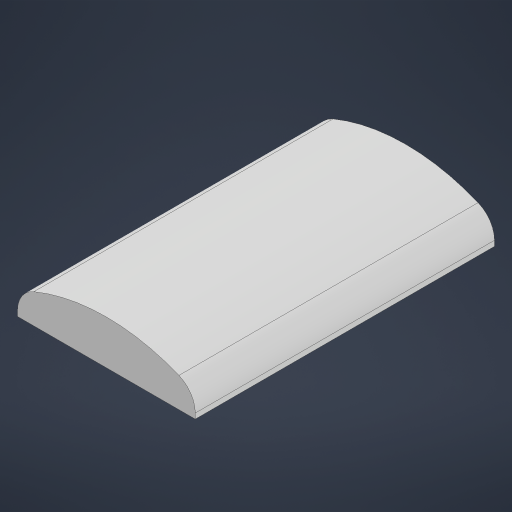
# Autodesk Inventor part: LED-streifen
Saved by Autodesk Inventor 2023 (Build 270158000, 158)
## iProperties
Created: 2022-04-28
Part Number: LED-streifen
Material: Generic
Document SubType Name: Modeling
Designer: Simon
Density: 1 g/cm^3
Appearance: Default
Author: Simon
Autodesk Inventor part; units mm, degrees
ref_plane "YZ Plane" through (0, 0, 0) normal (1, 0, 0) x (0, 1, 0)
ref_plane "XZ Plane" through (0, 0, 0) normal (0, 1, 0) x (-1, 0, 0)
ref_plane "XY Plane" through (0, 0, 0) normal (0, 0, 1) x (1, 0, 0)
sketch "Sketch1" plane through (0, 0, 0) normal (0, 1, 0) x (-1, 0, 0)
  line L0 (5.05, 8.5) -> (-5.05, 8.5)
  line L1 (-5.05, 8.5) -> (-5.05, -8.5)
  line L2 (-5.05, -8.5) -> (5.05, -8.5)
  line L3 (5.05, -8.5) -> (5.05, 8.5)
  line L4 (5.05, 8.5) -> (-5.05, -8.5) construction
  line L5 (-5.05, 8.5) -> (5.05, -8.5) construction
  point P0 (0, 0)
  dimension "d0" = 10.1
  dimension "d1" = 17
  constraints: 12 end point, 2 midpoint, 2 parallel, 1 horizontal, 1 perpendicular
  measures "d0" distance of L2.end L1.end
  measures "d1" distance of L1.end L0.end
extrude "Extrusion1" add sketch "Sketch1" along normal blind 2.5
sketch "Sketch2" plane through (-5.05, 0, 8.5) normal (0, 0, 1) x (1, 0, 0)
  line L0 (10.1, 0) -> (10.1, 2.5) projected
  line L1 (0, 0) -> (0, 2.5) projected
  arc A0 (10.1, 1.25) -> (0, 1.25) centre (5.05, -8.326) ccw
  line L2 (10.1, 0) -> (0, 0) projected
  line L3 (0, 0) -> (10.1, 0)
  line L4 (10.1, 0) -> (10.1, 1.25)
  point P0 (5.05, 0)
  constraints: 4 end point, 2 midpoint, 2 point on circle, 1 centre point, 1 perpendicular
extrude "Extrusion2" cut sketch "Sketch2" against normal blind 18.1375 keep common part
fillet "Fillet1" radius 1.5 2 edges at (-5.05, 1.25, 0) (5.05, 1.25, 0)
body "Solid1"
